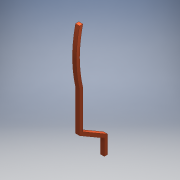
# Autodesk Inventor part: pins
Saved by Autodesk Inventor 2016 (Build 200138000, 138)
## iProperties
Created: 2016-07-08
Part Number: pins
Material: Copper
Document SubType Name: Modeling
Designer: Jonathan
Density: 8.94 g/cm^3
Appearance: Copper - Satin
Author: Jonathan
Autodesk Inventor part; units mm, degrees
ref_plane "YZ Plane" through (0, 0, 0) normal (1, 0, 0) x (0, 1, 0)
ref_plane "XZ Plane" through (0, 0, 0) normal (0, 1, 0) x (-1, 0, 0)
ref_plane "XY Plane" through (0, 0, 0) normal (0, 0, 1) x (1, 0, 0)
sketch "Sketch1" plane through (0, 0, 0) normal (1, 0, 0) x (0, 1, 0)
  line L0 (-1.75, 0.786) -> (-0.2, -0.1151)
  line L1 (-0.2, -0.1151) -> (-0.2, -1.1151)
  line L2 (-0.2, -1.1151) -> (0, -1.1151)
  line L3 (0, -1.1151) -> (0, 0)
  line L4 (0, 0) -> (-1.55, 0.901)
  line L5 (-1.55, 0.901) -> (-1.55, 3.3091)
  line L6 (-1.55, 6.75) -> (-1.7553, 6.75)
  line L7 (-1.75, 3.286) -> (-1.75, 0.786)
  arc A0 (-1.7553, 6.75) -> (-1.75, 3.286) centre (5.75, 5.0295) ccw
  arc A1 (-1.55, 6.75) -> (-1.55, 3.3091) centre (5.75, 5.0295) ccw
  line L8 (-1.95, 6.0295) -> (-1.95, 4.0295) construction
  point P0 (-0.1, -1.1151)
  point P1 (-1.6527, 6.75)
  point P2 (-1.95, 5.0295)
  dimension "d4" = 1
  dimension "d7" = 0.2
  dimension "d8" = 0.2
  dimension "d26" = 0.2
  dimension "d29" = 6.75
  dimension "d32" = 2
  dimension "d33" = 0.4
  dimension "d34" = 0.2
  dimension "d36" = 2.5
  dimension "d37" = 7.5
  dimension "d38" = 1.65
  constraints: 18 end point, 4 point on circle, 3 midpoint, 2 centre point, 2 parallel, 2 perpendicular, 1 coincident, 1 concentric, 1 horizontal, 1 horizontal alignment, 1 tangent, 1 vertical, 1 vertical alignment
  measures "d4" distance of L0.end L1.end
  measures "d7" distance between parallel lines of L0 L4
  measures "d8" distance between parallel lines of L3 L1
  measures "d26" distance between parallel lines of L5 L7
  measures "d29" distance from line of point (0, 0) L6
  measures "d32" distance of L8.start L8.end
  measures "d33" distance between parallel lines of L5 L8
  measures "d34" radial gap between concentric circles of A0 A1
  measures "d36" distance of L7.start L0.start
  measures "d37" radius of A1
  measures "d38" distance from line of point (-0.1, -1.115) L7
extrude "Extrusion1" add sketch "Sketch1" along normal mid plane 0.25
body "Solid1"
